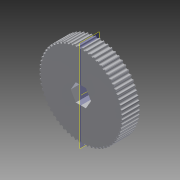
# Autodesk Inventor part: 64t Tooth Pulley .500 Hex Bore 3mm GT2
Saved by Autodesk Inventor 2013 (Build 170138000, 138)
## iProperties
Created: 2013-04-02
Part Number: 64t Tooth Pulley .500 Hex Bore 3mm GT2
Material: Generic
Document SubType Name: Modeling
Designer: mvarma
Density: 1 g/cm^3
Author: mvarma
Autodesk Inventor part; units mm, degrees
ref_plane "YZ Plane" through (0, 0, 0) normal (1, 0, 0) x (0, 1, 0)
ref_plane "XZ Plane" through (0, 0, 0) normal (0, 1, 0) x (-1, 0, 0)
sketch "Sketch1" plane through (0, 0, 0) normal (0, 0, 1) x (1, 0, 0)
  arc A0 (0.1766, -0.2413) -> (1.6659, -1.4291) centre (1.0365, -0.6906) ccw
  arc A1 (0.1766, -0.2413) -> (0.1766, 0.2413) centre (0, 0) ccw
  arc A2 (0.1766, 0.2413) -> (-0.1946, 0.5086) centre (-17.6567, -24.1311) ccw
  arc A3 (-0.1946, 0.5086) -> (-0.6523, 0.3556) centre (-0.3675, 0.2646) ccw
  arc A4 (-2.2509, 1.3916) -> (-0.6523, 0.3556) centre (-1.351, 1.0288) ccw
  arc A5 (-2.2509, 1.3916) -> (-2.2982, 1.8719) centre (-2.4503, 1.6145) ccw
  arc A6 (-2.2982, 1.8719) -> (-2.6938, 2.1015) centre (-17.6567, -24.1311) ccw
  arc A7 (-2.6938, 2.1015) -> (-3.1343, 1.9044) centre (-2.8419, 1.8418) ccw
  arc A8 (-4.8268, 2.7788) -> (-3.1343, 1.9044) centre (-3.8957, 2.5058) ccw
  arc A9 (-4.8268, 2.7788) -> (-4.9209, 3.2521) centre (-5.047, 2.981) ccw
  arc A10 (-4.9209, 3.2521) -> (-5.3371, 3.4418) centre (-17.6567, -24.1311) ccw
  arc A11 (-5.3371, 3.4418) -> (-5.7561, 3.2025) centre (-5.459, 3.1688) ccw
  arc A12 (-7.5262, 3.9067) -> (-5.7561, 3.2025) centre (-6.5728, 3.7264) ccw
  arc A13 (-7.5262, 3.9067) -> (-7.6663, 4.3686) centre (-7.7652, 4.0864) ccw
  arc A14 (-7.6663, 4.3686) -> (-8.099, 4.5166) centre (-17.6567, -24.1311) ccw
  arc A15 (-8.099, 4.5166) -> (-8.4926, 4.2373) centre (-8.1936, 4.233) ccw
  arc A16 (-10.3231, 4.7647) -> (-8.4926, 4.2373) centre (-9.3567, 4.6787) ccw
  arc A17 (-10.3231, 4.7647) -> (-10.5078, 5.2106) centre (-10.5786, 4.9201) ccw
  arc A18 (-10.5078, 5.2106) -> (-10.953, 5.3155) centre (-17.6567, -24.1311) ccw
  arc A19 (-10.953, 5.3155) -> (-11.3173, 4.999) centre (-11.0194, 5.0239) ccw
  arc A20 (-13.1907, 5.3444) -> (-11.3173, 4.999) centre (-12.2205, 5.3535) ccw
  arc A21 (-13.1907, 5.3444) -> (-13.4182, 5.77) centre (-13.4602, 5.4739) ccw
  arc A22 (-13.4182, 5.77) -> (-13.8715, 5.8307) centre (-17.6567, -24.1311) ccw
  arc A23 (-13.8715, 5.8307) -> (-14.2031, 5.4801) centre (-13.909, 5.5341) ccw
  arc A24 (-16.1014, 5.6402) -> (-14.2031, 5.4801) centre (-15.1367, 5.7444) ccw
  arc A25 (-16.1014, 5.6402) -> (-16.3695, 6.0414) centre (-16.3822, 5.7427) ccw
  arc A26 (-16.3695, 6.0414) -> (-16.8265, 6.0575) centre (-17.6567, -24.1311) ccw
  arc A27 (-16.8265, 6.0575) -> (-17.1221, 5.676) centre (-16.8348, 5.7586) ccw
  arc A28 (-19.0269, 5.6493) -> (-17.1221, 5.676) centre (-18.0771, 5.8475) ccw
  arc A29 (-19.0269, 5.6493) -> (-19.3331, 6.0223) centre (-19.3165, 5.7238) ccw
  arc A30 (-19.3331, 6.0223) -> (-19.7895, 5.9935) centre (-17.6567, -24.1311) ccw
  arc A31 (-19.7895, 5.9935) -> (-20.0463, 5.5848) centre (-19.7684, 5.6952) ccw
  arc A32 (-21.9393, 5.3716) -> (-20.0463, 5.5848) centre (-21.0135, 5.6619) ccw
  arc A33 (-21.9393, 5.3716) -> (-22.2806, 5.7128) centre (-22.2348, 5.4173) ccw
  arc A34 (-22.2806, 5.7128) -> (-22.732, 5.6394) centre (-17.6567, -24.1311) ccw
  arc A35 (-22.732, 5.6394) -> (-22.9475, 5.2075) centre (-22.6817, 5.3446) ccw
  arc A36 (-24.8105, 4.8097) -> (-22.9475, 5.2075) centre (-23.9176, 5.1895) ccw
  arc A37 (-24.8105, 4.8097) -> (-25.1835, 5.1159) centre (-25.109, 4.8263) ccw
  arc A38 (-25.1835, 5.1159) -> (-25.6256, 4.9986) centre (-17.6567, -24.1311) ccw
  arc A39 (-25.6256, 4.9986) -> (-25.7977, 4.5477) centre (-25.5467, 4.7101) ccw
  arc A40 (-27.6127, 3.9692) -> (-25.7977, 4.5477) centre (-26.7614, 4.4346) ccw
  arc A41 (-27.6127, 3.9692) -> (-28.014, 4.2373) centre (-27.9115, 3.9564) ccw
  arc A42 (-28.014, 4.2373) -> (-28.4424, 4.0772) centre (-17.6567, -24.1311) ccw
  arc A43 (-28.4424, 4.0772) -> (-28.5695, 3.6116) centre (-28.3356, 3.7979) ccw
  arc A44 (-30.3191, 2.858) -> (-28.5695, 3.6116) centre (-29.5174, 3.4046) ccw
  arc A45 (-30.3191, 2.858) -> (-30.7447, 3.0855) centre (-30.6151, 2.816) ccw
  arc A46 (-30.7447, 3.0855) -> (-31.1554, 2.8842) centre (-17.6567, -24.1311) ccw
  arc A47 (-31.1554, 2.8842) -> (-31.2362, 2.4084) centre (-31.0217, 2.6167) ccw
  arc A48 (-32.9035, 1.4869) -> (-31.2362, 2.4084) centre (-32.1593, 2.1095) ccw
  arc A49 (-32.9035, 1.4869) -> (-33.3494, 1.6716) centre (-33.194, 1.4161) ccw
  arc A50 (-33.3494, 1.6716) -> (-33.7383, 1.431) centre (-17.6567, -24.1311) ccw
  arc A51 (-33.7383, 1.431) -> (-33.7721, 0.9496) centre (-33.5791, 1.1779) ccw
  arc A52 (-35.3411, -0.1309) -> (-33.7721, 0.9496) centre (-34.6615, 0.5616) ccw
  arc A53 (-35.3411, -0.1309) -> (-35.8029, 0.0092) centre (-35.6233, -0.2298) ccw
  arc A54 (-35.8029, 0.0092) -> (-36.1664, -0.2684) centre (-17.6567, -24.1311) ccw
  arc A55 (-36.1664, -0.2684) -> (-36.1529, -0.7508) centre (-35.9832, -0.5046) ccw
  arc A56 (-37.6084, -1.9798) -> (-36.1529, -0.7508) centre (-36.9999, -1.224) ccw
  arc A57 (-37.6084, -1.9798) -> (-38.0817, -1.8857) centre (-37.8795, -2.1059) ccw
  arc A58 (-38.0817, -1.8857) -> (-38.4162, -2.1975) centre (-17.6567, -24.1311) ccw
  arc A59 (-38.4162, -2.1975) -> (-38.3555, -2.6763) centre (-38.2107, -2.4147) ccw
  arc A60 (-39.6835, -4.0421) -> (-38.3555, -2.6763) centre (-39.1521, -3.2303) ccw
  arc A61 (-39.6835, -4.0421) -> (-40.1638, -3.9948) centre (-39.941, -4.1942) ccw
  arc A62 (-40.1638, -3.9948) -> (-40.4662, -4.3379) centre (-17.6567, -24.1311) ccw
  arc A63 (-40.4662, -4.3379) -> (-40.3588, -4.8085) centre (-40.2403, -4.5339) ccw
  arc A64 (-41.5465, -6.2978) -> (-40.3588, -4.8085) centre (-41.0972, -5.4379) ccw
  arc A65 (-41.5465, -6.2978) -> (-42.0291, -6.2978) centre (-41.7878, -6.4744) ccw
  arc A66 (-42.0291, -6.2978) -> (-42.2964, -6.669) centre (-17.6567, -24.1311) ccw
  arc A67 (-42.2964, -6.669) -> (-42.1434, -7.1267) centre (-42.0524, -6.8419) ccw
  arc A68 (-43.1794, -8.7253) -> (-42.1434, -7.1267) centre (-42.8166, -7.8254) ccw
  arc A69 (-43.1794, -8.7253) -> (-43.6597, -8.7726) centre (-43.4023, -8.9247) ccw
  arc A70 (-43.6597, -8.7726) -> (-43.8893, -9.1682) centre (-17.6567, -24.1311) ccw
  arc A71 (-43.8893, -9.1682) -> (-43.6922, -9.6087) centre (-43.6296, -9.3163) ccw
  arc A72 (-44.5666, -11.3012) -> (-43.6922, -9.6087) centre (-44.2937, -10.3701) ccw
  arc A73 (-44.5666, -11.3012) -> (-45.0399, -11.3953) centre (-44.7688, -11.5214) ccw
  arc A74 (-45.0399, -11.3953) -> (-45.2296, -11.8115) centre (-17.6567, -24.1311) ccw
  arc A75 (-45.2296, -11.8115) -> (-44.9903, -12.2305) centre (-44.9566, -11.9334) ccw
  arc A76 (-45.6946, -14.0006) -> (-44.9903, -12.2305) centre (-45.5142, -13.0472) ccw
  arc A77 (-45.6946, -14.0006) -> (-46.1564, -14.1407) centre (-45.8742, -14.2396) ccw
  arc A78 (-46.1564, -14.1407) -> (-46.3044, -14.5734) centre (-17.6567, -24.1311) ccw
  arc A79 (-46.3044, -14.5734) -> (-46.0251, -14.967) centre (-46.0208, -14.668) ccw
  arc A80 (-46.5525, -16.7975) -> (-46.0251, -14.967) centre (-46.4665, -15.8311) ccw
  arc A81 (-46.5525, -16.7975) -> (-46.9984, -16.9822) centre (-46.7079, -17.053) ccw
  arc A82 (-46.9984, -16.9822) -> (-47.1033, -17.4274) centre (-17.6567, -24.1311) ccw
  arc A83 (-47.1033, -17.4274) -> (-46.7868, -17.7917) centre (-46.8117, -17.4938) ccw
  arc A84 (-47.1322, -19.6651) -> (-46.7868, -17.7917) centre (-47.1413, -18.6949) ccw
  arc A85 (-47.1322, -19.6651) -> (-47.5578, -19.8926) centre (-47.2618, -19.9346) ccw
  arc A86 (-47.5578, -19.8926) -> (-47.6186, -20.3459) centre (-17.6567, -24.1311) ccw
  arc A87 (-47.6186, -20.3459) -> (-47.2679, -20.6775) centre (-47.3219, -20.3834) ccw
  arc A88 (-47.428, -22.5758) -> (-47.2679, -20.6775) centre (-47.5322, -21.6111) ccw
  arc A89 (-47.428, -22.5758) -> (-47.8293, -22.8439) centre (-47.5305, -22.8566) ccw
  arc A90 (-47.8293, -22.8439) -> (-47.8453, -23.3009) centre (-17.6567, -24.1311) ccw
  arc A91 (-47.8453, -23.3009) -> (-47.4638, -23.5965) centre (-47.5464, -23.3092) ccw
  arc A92 (-47.4371, -25.5013) -> (-47.4638, -23.5965) centre (-47.6353, -24.5515) ccw
  arc A93 (-47.4371, -25.5013) -> (-47.8101, -25.8075) centre (-47.5116, -25.7909) ccw
  arc A94 (-47.8101, -25.8075) -> (-47.7813, -26.2639) centre (-17.6567, -24.1311) ccw
  arc A95 (-47.7813, -26.2639) -> (-47.3727, -26.5207) centre (-47.483, -26.2428) ccw
  arc A96 (-47.1594, -28.4137) -> (-47.3727, -26.5207) centre (-47.4498, -27.4879) ccw
  arc A97 (-47.1594, -28.4137) -> (-47.5006, -28.755) centre (-47.2052, -28.7092) ccw
  arc A98 (-47.5006, -28.755) -> (-47.4272, -29.2064) centre (-17.6567, -24.1311) ccw
  arc A99 (-47.4272, -29.2064) -> (-46.9954, -29.4219) centre (-47.1324, -29.1561) ccw
  arc A100 (-46.5975, -31.2849) -> (-46.9954, -29.4219) centre (-46.9773, -30.392) ccw
  arc A101 (-46.5975, -31.2849) -> (-46.9037, -31.6579) centre (-46.6141, -31.5834) ccw
  arc A102 (-46.9037, -31.6579) -> (-46.7864, -32.1) centre (-17.6567, -24.1311) ccw
  arc A103 (-46.7864, -32.1) -> (-46.3355, -32.2721) centre (-46.498, -32.0211) ccw
  arc A104 (-45.757, -34.0871) -> (-46.3355, -32.2721) centre (-46.2224, -33.2358) ccw
  arc A105 (-45.757, -34.0871) -> (-46.0251, -34.4884) centre (-45.7443, -34.3859) ccw
  arc A106 (-46.0251, -34.4884) -> (-45.865, -34.9168) centre (-17.6567, -24.1311) ccw
  arc A107 (-45.865, -34.9168) -> (-45.3994, -35.0439) centre (-45.5857, -34.81) ccw
  arc A108 (-44.6458, -36.7935) -> (-45.3994, -35.0439) centre (-45.1924, -35.9918) ccw
  arc A109 (-44.6458, -36.7935) -> (-44.8733, -37.2191) centre (-44.6039, -37.0895) ccw
  arc A110 (-44.8733, -37.2191) -> (-44.672, -37.6298) centre (-17.6567, -24.1311) ccw
  arc A111 (-44.672, -37.6298) -> (-44.1962, -37.7106) centre (-44.4045, -37.4961) ccw
  arc A112 (-43.2747, -39.3779) -> (-44.1962, -37.7106) centre (-43.8973, -38.6337) ccw
  arc A113 (-43.2747, -39.3779) -> (-43.4594, -39.8238) centre (-43.204, -39.6684) ccw
  arc A114 (-43.4594, -39.8238) -> (-43.2188, -40.2127) centre (-17.6567, -24.1311) ccw
  arc A115 (-43.2188, -40.2127) -> (-42.7374, -40.2466) centre (-42.9657, -40.0535) ccw
  arc A116 (-41.6569, -41.8155) -> (-42.7374, -40.2466) centre (-42.3494, -41.1359) ccw
  arc A117 (-41.6569, -41.8155) -> (-41.797, -42.2773) centre (-41.558, -42.0977) ccw
  arc A118 (-41.797, -42.2773) -> (-41.5195, -42.6408) centre (-17.6567, -24.1311) ccw
  arc A119 (-41.5195, -42.6408) -> (-41.037, -42.6273) centre (-41.2832, -42.4576) ccw
  arc A120 (-39.808, -44.0828) -> (-41.037, -42.6273) centre (-40.5638, -43.4743) ccw
  arc A121 (-39.808, -44.0828) -> (-39.9021, -44.5561) centre (-39.6819, -44.3539) ccw
  arc A122 (-39.9021, -44.5561) -> (-39.5903, -44.8906) centre (-17.6567, -24.1311) ccw
  arc A123 (-39.5903, -44.8906) -> (-39.1115, -44.8299) centre (-39.3731, -44.6851) ccw
  arc A124 (-37.7457, -46.1579) -> (-39.1115, -44.8299) centre (-38.5575, -45.6265) ccw
  arc A125 (-37.7457, -46.1579) -> (-37.793, -46.6382) centre (-37.5937, -46.4154) ccw
  arc A126 (-37.793, -46.6382) -> (-37.4499, -46.9406) centre (-17.6567, -24.1311) ccw
  arc A127 (-37.4499, -46.9406) -> (-36.9794, -46.8332) centre (-37.2539, -46.7147) ccw
  arc A128 (-35.49, -48.0209) -> (-36.9794, -46.8332) centre (-36.35, -47.5716) ccw
  arc A129 (-35.49, -48.0209) -> (-35.49, -48.5035) centre (-35.3134, -48.2622) ccw
  arc A130 (-35.49, -48.5035) -> (-35.1188, -48.7708) centre (-17.6567, -24.1311) ccw
  arc A131 (-35.1188, -48.7708) -> (-34.6611, -48.6178) centre (-34.946, -48.5268) ccw
  arc A132 (-33.0625, -49.6538) -> (-34.6611, -48.6178) centre (-33.9624, -49.291) ccw
  arc A133 (-33.0625, -49.6538) -> (-33.0152, -50.1341) centre (-32.8631, -49.8767) ccw
  arc A134 (-33.0152, -50.1341) -> (-32.6197, -50.3637) centre (-17.6567, -24.1311) ccw
  arc A135 (-32.6197, -50.3637) -> (-32.1791, -50.1666) centre (-32.4715, -50.104) ccw
  arc A136 (-30.4866, -51.041) -> (-32.1791, -50.1666) centre (-31.4178, -50.7681) ccw
  arc A137 (-30.4866, -51.041) -> (-30.3925, -51.5143) centre (-30.2664, -51.2432) ccw
  arc A138 (-30.3925, -51.5143) -> (-29.9764, -51.704) centre (-17.6567, -24.1311) ccw
  arc A139 (-29.9764, -51.704) -> (-29.5573, -51.4647) centre (-29.8544, -51.431) ccw
  arc A140 (-27.7872, -52.169) -> (-29.5573, -51.4647) centre (-28.7406, -51.9886) ccw
  arc A141 (-27.7872, -52.169) -> (-27.6471, -52.6308) centre (-27.5482, -52.3486) ccw
  arc A142 (-27.6471, -52.6308) -> (-27.2144, -52.7788) centre (-17.6567, -24.1311) ccw
  arc A143 (-27.2144, -52.7788) -> (-26.8208, -52.4995) centre (-27.1198, -52.4952) ccw
  arc A144 (-24.9903, -53.0269) -> (-26.8208, -52.4995) centre (-25.9567, -52.9409) ccw
  arc A145 (-24.9903, -53.0269) -> (-24.8056, -53.4728) centre (-24.7348, -53.1823) ccw
  arc A146 (-24.8056, -53.4728) -> (-24.3604, -53.5777) centre (-17.6567, -24.1311) ccw
  arc A147 (-24.3604, -53.5777) -> (-23.9961, -53.2612) centre (-24.2941, -53.2861) ccw
  arc A148 (-22.1227, -53.6066) -> (-23.9961, -53.2612) centre (-23.0929, -53.6157) ccw
  arc A149 (-22.1227, -53.6066) -> (-21.8952, -54.0322) centre (-21.8532, -53.7362) ccw
  arc A150 (-21.8952, -54.0322) -> (-21.4419, -54.093) centre (-17.6567, -24.1311) ccw
  arc A151 (-21.4419, -54.093) -> (-21.1103, -53.7423) centre (-21.4044, -53.7963) ccw
  arc A152 (-19.2121, -53.9024) -> (-21.1103, -53.7423) centre (-20.1767, -54.0066) ccw
  arc A153 (-19.2121, -53.9024) -> (-18.9439, -54.3037) centre (-18.9312, -54.0049) ccw
  arc A154 (-18.9439, -54.3037) -> (-18.4869, -54.3197) centre (-17.6567, -24.1311) ccw
  arc A155 (-18.4869, -54.3197) -> (-18.1913, -53.9382) centre (-18.4787, -54.0208) ccw
  arc A156 (-16.2865, -53.9115) -> (-18.1913, -53.9382) centre (-17.2363, -54.1097) ccw
  arc A157 (-16.2865, -53.9115) -> (-15.9803, -54.2845) centre (-15.9969, -53.986) ccw
  arc A158 (-15.9803, -54.2845) -> (-15.5239, -54.2557) centre (-17.6567, -24.1311) ccw
  arc A159 (-15.5239, -54.2557) -> (-15.2671, -53.8471) centre (-15.545, -53.9574) ccw
  arc A160 (-13.3741, -53.6338) -> (-15.2671, -53.8471) centre (-14.2999, -53.9242) ccw
  arc A161 (-13.3741, -53.6338) -> (-13.0328, -53.975) centre (-13.0786, -53.6796) ccw
  arc A162 (-13.0328, -53.975) -> (-12.5814, -53.9016) centre (-17.6567, -24.1311) ccw
  arc A163 (-12.5814, -53.9016) -> (-12.3659, -53.4698) centre (-12.6317, -53.6068) ccw
  arc A164 (-10.5029, -53.0719) -> (-12.3659, -53.4698) centre (-11.3958, -53.4517) ccw
  arc A165 (-10.5029, -53.0719) -> (-10.1299, -53.3781) centre (-10.2044, -53.0885) ccw
  arc A166 (-10.1299, -53.3781) -> (-9.6878, -53.2608) centre (-17.6567, -24.1311) ccw
  arc A167 (-9.6878, -53.2608) -> (-9.5157, -52.8099) centre (-9.7667, -52.9724) ccw
  arc A168 (-7.7007, -52.2314) -> (-9.5157, -52.8099) centre (-8.5521, -52.6968) ccw
  arc A169 (-7.7007, -52.2314) -> (-7.2994, -52.4995) centre (-7.402, -52.2187) ccw
  arc A170 (-7.2994, -52.4995) -> (-6.871, -52.3394) centre (-17.6567, -24.1311) ccw
  arc A171 (-6.871, -52.3394) -> (-6.7439, -51.8738) centre (-6.9778, -52.0601) ccw
  arc A172 (-4.9943, -51.1202) -> (-6.7439, -51.8738) centre (-5.796, -51.6668) ccw
  arc A173 (-4.9943, -51.1202) -> (-4.5687, -51.3477) centre (-4.6983, -51.0783) ccw
  arc A174 (-4.5687, -51.3477) -> (-4.158, -51.1464) centre (-17.6567, -24.1311) ccw
  arc A175 (-4.158, -51.1464) -> (-4.0772, -50.6706) centre (-4.2917, -50.8789) ccw
  arc A176 (-2.4099, -49.7491) -> (-4.0772, -50.6706) centre (-3.1541, -50.3717) ccw
  arc A177 (-2.4099, -49.7491) -> (-1.964, -49.9338) centre (-2.1194, -49.6784) ccw
  arc A178 (-1.964, -49.9338) -> (-1.5751, -49.6932) centre (-17.6567, -24.1311) ccw
  arc A179 (-1.5751, -49.6932) -> (-1.5413, -49.2118) centre (-1.7343, -49.4401) ccw
  arc A180 (0.0277, -48.1313) -> (-1.5413, -49.2118) centre (-0.6519, -48.8238) ccw
  arc A181 (0.0277, -48.1313) -> (0.4895, -48.2714) centre (0.3099, -48.0324) ccw
  arc A182 (0.4895, -48.2714) -> (0.853, -47.9939) centre (-17.6567, -24.1311) ccw
  arc A183 (0.853, -47.9939) -> (0.8395, -47.5114) centre (0.6697, -47.7576) ccw
  arc A184 (2.295, -46.2824) -> (0.8395, -47.5114) centre (1.6865, -47.0382) ccw
  arc A185 (2.295, -46.2824) -> (2.7683, -46.3765) centre (2.5661, -46.1563) ccw
  arc A186 (2.7683, -46.3765) -> (3.1028, -46.0647) centre (-17.6567, -24.1311) ccw
  arc A187 (3.1028, -46.0647) -> (3.0421, -45.5859) centre (2.8973, -45.8475) ccw
  arc A188 (4.3701, -44.2201) -> (3.0421, -45.5859) centre (3.8386, -45.0319) ccw
  arc A189 (4.3701, -44.2201) -> (4.8504, -44.2674) centre (4.6275, -44.0681) ccw
  arc A190 (4.8504, -44.2674) -> (5.1527, -43.9243) centre (-17.6567, -24.1311) ccw
  arc A191 (5.1527, -43.9243) -> (5.0453, -43.4538) centre (4.9269, -43.7283) ccw
  arc A192 (6.2331, -41.9644) -> (5.0453, -43.4538) centre (5.7838, -42.8244) ccw
  arc A193 (6.2331, -41.9644) -> (6.7157, -41.9644) centre (6.4744, -41.7878) ccw
  arc A194 (6.7157, -41.9644) -> (6.983, -41.5932) centre (-17.6567, -24.1311) ccw
  arc A195 (6.983, -41.5932) -> (6.83, -41.1355) centre (6.739, -41.4204) ccw
  arc A196 (7.866, -39.5369) -> (6.83, -41.1355) centre (7.5032, -40.4368) ccw
  arc A197 (7.866, -39.5369) -> (8.3463, -39.4896) centre (8.0889, -39.3375) ccw
  arc A198 (8.3463, -39.4896) -> (8.5759, -39.0941) centre (-17.6567, -24.1311) ccw
  arc A199 (8.5759, -39.0941) -> (8.3788, -38.6535) centre (8.3162, -38.9459) ccw
  arc A200 (9.2532, -36.961) -> (8.3788, -38.6535) centre (8.9802, -37.8922) ccw
  arc A201 (9.2532, -36.961) -> (9.7265, -36.8669) centre (9.4554, -36.7408) ccw
  arc A202 (9.7265, -36.8669) -> (9.9162, -36.4508) centre (-17.6567, -24.1311) ccw
  arc A203 (9.9162, -36.4508) -> (9.6769, -36.0317) centre (9.6432, -36.3288) ccw
  arc A204 (10.3811, -34.2616) -> (9.6769, -36.0317) centre (10.2008, -35.215) ccw
  arc A205 (10.3811, -34.2616) -> (10.843, -34.1215) centre (10.5608, -34.0226) ccw
  arc A206 (10.843, -34.1215) -> (10.991, -33.6888) centre (-17.6567, -24.1311) ccw
  arc A207 (10.991, -33.6888) -> (10.7117, -33.2952) centre (10.7074, -33.5942) ccw
  arc A208 (11.2391, -31.4647) -> (10.7117, -33.2952) centre (11.1531, -32.4311) ccw
  arc A209 (11.2391, -31.4647) -> (11.685, -31.28) centre (11.3945, -31.2092) ccw
  arc A210 (11.685, -31.28) -> (11.7899, -30.8348) centre (-17.6567, -24.1311) ccw
  arc A211 (11.7899, -30.8348) -> (11.4734, -30.4705) centre (11.4983, -30.7685) ccw
  arc A212 (11.8188, -28.5971) -> (11.4734, -30.4705) centre (11.8279, -29.5673) ccw
  arc A213 (11.8188, -28.5971) -> (12.2444, -28.3696) centre (11.9483, -28.3276) ccw
  arc A214 (12.2444, -28.3696) -> (12.3051, -27.9163) centre (-17.6567, -24.1311) ccw
  arc A215 (12.3051, -27.9163) -> (11.9545, -27.5847) centre (12.0085, -27.8788) ccw
  arc A216 (12.1146, -25.6865) -> (11.9545, -27.5847) centre (12.2188, -26.6511) ccw
  arc A217 (12.1146, -25.6865) -> (12.5158, -25.4183) centre (12.2171, -25.4056) ccw
  arc A218 (12.5158, -25.4183) -> (12.5319, -24.9613) centre (-17.6567, -24.1311) ccw
  arc A219 (12.5319, -24.9613) -> (12.1504, -24.6657) centre (12.233, -24.9531) ccw
  arc A220 (12.1237, -22.7609) -> (12.1504, -24.6657) centre (12.3219, -23.7107) ccw
  arc A221 (12.1237, -22.7609) -> (12.4967, -22.4547) centre (12.1982, -22.4713) ccw
  arc A222 (12.4967, -22.4547) -> (12.4679, -21.9983) centre (-17.6567, -24.1311) ccw
  arc A223 (12.4679, -21.9983) -> (12.0592, -21.7415) centre (12.1696, -22.0194) ccw
  arc A224 (11.846, -19.8485) -> (12.0592, -21.7415) centre (12.1363, -20.7743) ccw
  arc A225 (11.846, -19.8485) -> (12.1872, -19.5072) centre (11.8917, -19.553) ccw
  arc A226 (12.1872, -19.5072) -> (12.1138, -19.0558) centre (-17.6567, -24.1311) ccw
  arc A227 (12.1138, -19.0558) -> (11.6819, -18.8403) centre (11.819, -19.1061) ccw
  arc A228 (11.2841, -16.9773) -> (11.6819, -18.8403) centre (11.6639, -17.8702) ccw
  arc A229 (11.2841, -16.9773) -> (11.5903, -16.6043) centre (11.3007, -16.6788) ccw
  arc A230 (11.5903, -16.6043) -> (11.473, -16.1622) centre (-17.6567, -24.1311) ccw
  arc A231 (11.473, -16.1622) -> (11.0221, -15.9901) centre (11.1845, -16.2411) ccw
  arc A232 (10.4436, -14.1751) -> (11.0221, -15.9901) centre (10.909, -15.0265) ccw
  arc A233 (10.4436, -14.1751) -> (10.7117, -13.7738) centre (10.4308, -13.8764) ccw
  arc A234 (10.7117, -13.7738) -> (10.5516, -13.3454) centre (-17.6567, -24.1311) ccw
  arc A235 (10.5516, -13.3454) -> (10.086, -13.2183) centre (10.2723, -13.4522) ccw
  arc A236 (9.3324, -11.4687) -> (10.086, -13.2183) centre (9.879, -12.2704) ccw
  arc A237 (9.3324, -11.4687) -> (9.5599, -11.0431) centre (9.2904, -11.1727) ccw
  arc A238 (9.5599, -11.0431) -> (9.3586, -10.6324) centre (-17.6567, -24.1311) ccw
  arc A239 (9.3586, -10.6324) -> (8.8828, -10.5516) centre (9.0911, -10.7661) ccw
  arc A240 (7.9613, -8.8843) -> (8.8828, -10.5516) centre (8.5839, -9.6285) ccw
  arc A241 (7.9613, -8.8843) -> (8.146, -8.4384) centre (7.8905, -8.5938) ccw
  arc A242 (8.146, -8.4384) -> (7.9054, -8.0495) centre (-17.6567, -24.1311) ccw
  arc A243 (7.9054, -8.0495) -> (7.424, -8.0157) centre (7.6523, -8.2087) ccw
  arc A244 (6.3435, -6.4467) -> (7.424, -8.0157) centre (7.036, -7.1263) ccw
  arc A245 (6.3435, -6.4467) -> (6.4836, -5.9849) centre (6.2446, -6.1645) ccw
  arc A246 (6.4836, -5.9849) -> (6.206, -5.6214) centre (-17.6567, -24.1311) ccw
  arc A247 (6.206, -5.6214) -> (5.7236, -5.6349) centre (5.9698, -5.8047) ccw
  arc A248 (4.4946, -4.1794) -> (5.7236, -5.6349) centre (5.2504, -4.7879) ccw
  arc A249 (4.4946, -4.1794) -> (4.5887, -3.7061) centre (4.3685, -3.9083) ccw
  arc A250 (4.5887, -3.7061) -> (4.2769, -3.3716) centre (-17.6567, -24.1311) ccw
  arc A251 (4.2769, -3.3716) -> (3.7981, -3.4323) centre (4.0597, -3.5771) ccw
  arc A252 (2.4323, -2.1043) -> (3.7981, -3.4323) centre (3.2441, -2.6358) ccw
  arc A253 (2.4323, -2.1043) -> (2.4796, -1.624) centre (2.2802, -1.8469) ccw
  arc A254 (2.4796, -1.624) -> (2.1365, -1.3217) centre (-17.6567, -24.1311) ccw
  arc A255 (2.1365, -1.3217) -> (1.6659, -1.4291) centre (1.9405, -1.5475) ccw
  line L0 (-24.9891, -24.1311) -> (-21.3229, -17.7811)
  line L1 (-21.3229, -17.7811) -> (-13.9905, -17.7811)
  line L2 (-13.9905, -17.7811) -> (-10.3244, -24.1311)
  line L3 (-10.3244, -24.1311) -> (-13.9905, -30.4811)
  line L4 (-13.9905, -30.4811) -> (-21.3229, -30.4811)
  line L5 (-21.3229, -30.4811) -> (-24.9891, -24.1311)
  circle A256 centre (-17.6567, -24.1311) radius 30.55 construction
  dimension "d2" = 12.7
  dimension "d3" = 61.1
  constraints: 512 point on circle, 257 centre point, 12 end point, 2 coincident, 1 horizontal, 782 other
  measures "d2" distance between parallel lines of L4 L1
  measures "d3" diameter of A256
extrude "Extrusion1" add sketch "Sketch1" along normal blind 12.7
ref_plane "Work Plane1" through (0, 0, 6.35) normal (0, 0, 1) x (1, 0, 0)
ref_plane "Work Plane2" through (-17.6567, -24.1311, 0) normal (-1, 0, 0) x (0, 0, 1)
body "Solid1"
